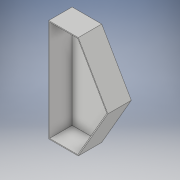
# Autodesk Inventor part: Half Hexagon Test v1
Saved by Autodesk Inventor 2019 (Build 230136000, 136)
## iProperties
Created: 2021-08-21
Part Number: Half Hexagon Test v1
Material: Generic
Document SubType Name: Modeling
Designer: Lix
Density: 1 g/cm^3
Appearance: Default
Author: Lix
Autodesk Inventor part; units mm, degrees
ref_plane "YZ Plane" through (0, 0, 0) normal (1, 0, 0) x (0, 1, 0)
ref_plane "XZ Plane" through (0, 0, 0) normal (0, 1, 0) x (-1, 0, 0)
ref_plane "XY Plane" through (0, 0, 0) normal (0, 0, 1) x (1, 0, 0)
sketch "Sketch1" plane through (0, 0, 0) normal (0, 0, 1) x (1, 0, 0)
  line L0 (50.5181, -87.5) -> (0, -87.5)
  line L1 (0, 87.5) -> (50.5181, 87.5)
  line L2 (50.5181, 87.5) -> (101.0363, 0)
  line L3 (101.0363, 0) -> (50.5181, -87.5)
  line L4 (0, 87.5) -> (0, -87.5)
  point P0 (0, 0)
  point P1 (0, 0)
  constraints: 10 end point, 1 coincident, 1 horizontal, 6 other
extrude "Extrusion1" add sketch "Sketch1" along normal blind 40
shell "Shell1" thickness 1.5 removed faces 1 at (33.6788, 0, 40)
body "Solid1"
